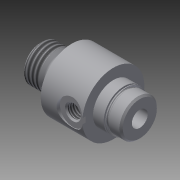
# Autodesk Inventor part: 01R000-0_rod_guide
Saved by Autodesk Inventor 2015 (Build 190159000, 159)
## iProperties
Category: PARTsolutions
Company: BIMBA
Created: 2015-01-25
Part Number: 01R000-0_rod_guide
Material: Generic
Catalog Web Link: www.cadenas.de
Description: Rod Guide-Original Line - Standard Air Cylinders
Vendor: BIMBA
Document SubType Name: Standard Catalog Part
Designer: whitaus15
Manufacturer: BIMBA
Mass: 4.50765 g
Surface Area: 24.6874 cm^2
Volume: 4.50765 cm^3
Density: 1 g/cm^3
Appearance: PSOLRGB-211-211-211
PSOL_IDENT_0: {$CADENAS_DATA\23d-libs\bimba\bimba\bimba_imperial\bimba_full_line\original_line_cylinders\standard_
PSOL_IDENT_1: air_cylinders\rod_guide.prj},232 {VTYP=3D},{NB=01R000-0_rod_guide},{LINA=01R000-0_rod_guide},{NN=Rod
PSOL_IDENT_2: Guide},{DATE=05.09.2013 09:10:53},{GEOMDATE=05.09.2013 11:10:00},{VERSION=},{LINEID=20},{LINESUBID=
PSOL_IDENT_3: -1},{WBVAR=MNT,ACTING,NR,K,Q,T1,T2,T3,T4,MB,TRIM,CUSH,RODTRANS}  {NB=01R000-0_rod_guide},{LINA=01R00
PSOL_IDENT_4: 0-0_rod_guide},{KT=DUMMY},{PN=01R000},{BORE=0.43750000},{BOREPN=01},{MNT=},{MNTALG='' , 'Front Nose'
PSOL_IDENT_5: , 'BF' , 'Front Block' , 'BFT' , 'Front Trunnion'},{ACTING=R},{ACTINGALG= '' , 'Single Acting' , 'R'
PSOL_IDENT_6: , 'Reverse/Double Acting' },{NR=},{NRALG= '' , 'N/A' },{K=},{Q=},{QALG= '' , 'Without Side Ported R
PSOL_IDENT_7: ear Head' , 'Q' , 'With Side Ported Rear Head' },{T1=},{T2=},{T3=},{T4=},{MB=0},{A1=1.1880},{A1N=0.6
PSOL_IDENT_8: 880},{A1P=1.1880},{A1B=1.1880},{A2=0.3750},{A2N=0.3130},{A2P=0.3750},{A3=0.6250},{A3N=0.1250},{A3P=0
PSOL_IDENT_9: .6250},{A4=0.1880},{A4N=0.2500},{A4P=0.1880},{A5=0.0200},{A6=0.0000},{A6N=0.0620},{A6P=0.0000},{A7=0
PSOL_IDENT_10: .5940},{A7N=0.1880},{A7P=0.5940},{A8=0.0200},{A8N=0.0200},{A8NR=0.0200},{D1=0.7380},{D1N=0.4840},{D1
PSOL_IDENT_11: P=0.7380},{D1B=0.0000},{D2=0.4465},{D3=0.0000},{D3N=0.3470},{D3P=0.0000},{D4=0.2820},{D4N=0.2220},{D
PSOL_IDENT_12: 4P=0.2820},{D4NR=0.2820},{D5=0.1895},{D5N=0.1895},{D5NR=0.1895},{C1=0.000},{C2=0.0200},{C2N=0.0200},
PSOL_IDENT_13: {C2P=0.0200},{C3=0.0000},{C3N=0.0000},{C3P=0.0000},{C4=0.0000},{C4N=0.0000},{C4P=0.0000},{NDM=0.4375
PSOL_IDENT_14: },{NDMN=0.3750},{NDMP=0.4375},{TAB=UNF},{D6=0.4350},{D6N=0.3725},{D6P=0.4350},{A9=0.0475},{A9N=0.050
PSOL_IDENT_15: 0},{A9P=0.0475},{D7=0.3600},{D7N=0.3100},{D7P=0.3600},{A10=0.0775},{A10N=0.0655},{A10P=0.0775},{R1=0
PSOL_IDENT_16: .0315},{R1N=0.0265},{R1P=0.0315},{D8=0.0000},{D9=0.0000},{D10=0.0000},{A11=0.0000},{A12=0.0000},{A13=
PSOL_IDENT_17: 0.0000},{A14=0.4680},{A14N=0.4680},{A14B=0.4690},{D11=0.0000},{D11N=0.0000},{NDM2=0.1900},{NDM2N=0.1
PSOL_IDENT_18: 900},{NDM2DP=0.0000},{THREAD=0},{HEX=0.1920},{HEXN=0.1920},{S1=0.7500},{B1=0.1275},{B2=0.3120},{B22=
PSOL_IDENT_19: 0.4380},{DB=0.3020},{B3=0.2200},{B4=0.4380},{X1=0.0620},{X2=0.4345},{NDM3=0.1640},{NDM4=0.1640},{NDM
PSOL_IDENT_20: 4DP=0.2500},{DD=0.7500},{CB=0.0000},{CBDP=0.0000},{PORT=1},{XT=0.3120},{XTX=0.3120},{XT1=0.3740},{XT
PSOL_IDENT_21: 2=0.2500},{NDMH=0.0000},{OD=0.4855},{ID=0.4465},{G=0.0000},{PNUT=0.3275},{TRIM=0},{C11=0.0000},{C22=
PSOL_IDENT_22: 0.0000},{C33=0.0000},{C44=0.0000},{C55=0.0000},{CD1=0.0000},{CD2=0.0000},{CD3=0.0000},{CNDM3=0.0000}
PSOL_IDENT_23: ,{CTAB3=0.0000},{CUSH=0},{XX=0.43800},{LCD=0.0000},{RODTRANS=0.00000}
NN: Rod Guide
NT: Original Line - Standard Air Cylinders
NB: 01R000-0_rod_guide
NBSYN: $PN.-$RODTRANS._rod_guide
LINA: 01R000-0_rod_guide
BORE: 7/16
BOREPN: 01
MNT: Front Nose
MNTALG: '' , 'Front Nose' , 'BF' , 'Front Block' , 'BFT' , 'Front Trunnion'
ACTING: Reverse/Double Acting
NR: N/A
K: Standard
Q: Without Side Ported Rear Head
T1: without T1
T2: without T2
T3: without T3
T4: without T4
MB: 0
A1N: 0.6880
A1P: 1.1880
A1B: 1.1880
A2N: 0.3130
A2P: 0.3750
A3N: 0.1250
A3P: 0.6250
A4N: 0.2500
A4P: 0.1880
A5: 0.0200
A6N: 0.0620
A6P: 0.0000
A7N: 0.1880
A7P: 0.5940
A8N: 0.0200
A8NR: 0.0200
D1N: 0.4840
D1P: 0.7380
D1B: 0.0000
D2: 0.4465
D3N: 0.3470
D3P: 0.0000
D4N: 0.2220
D4P: 0.2820
D4NR: 0.2820
D5N: 0.1895
D5NR: 0.1895
C1: 0.000
C2N: 0.0200
C2P: 0.0200
C3N: 0.0000
C3P: 0.0000
C4N: 0.0000
C4P: 0.0000
NDMN: 0.3750
NDMP: 0.4375
TAB: UNF
D6N: 0.3725
D6P: 0.4350
A9N: 0.0500
A9P: 0.0475
D7N: 0.3100
D7P: 0.3600
A10N: 0.0655
A10P: 0.0775
R1N: 0.0265
R1P: 0.0315
D8: 0.0000
D9: 0.0000
D10: 0.0000
A11: 0.0000
A12: 0.0000
A13: 0.0000
A14N: 0.4680
A14B: 0.4690
D11N: 0.0000
NDM2N: 0.1900
NDM2DP: 0.0000
HEXN: 0.1920
S1: 0.7500
B1: 0.1275
B2: 0.3120
B22: 0.4380
DB: 0.3020
B3: 0.2200
B4: 0.4380
X1: 0.0620
X2: 0.4345
NDM3: 0.1640
NDM4: 0.1640
NDM4DP: 0.2500
DD: 0.7500
CB: 0.0000
CBDP: 0.0000
XTX: 0.3120
XT1: 0.3740
XT2: 0.2500
NDMH: 0.0000
TRIM: 0
C11: 0.0000
C22: 0.0000
C33: 0.0000
C44: 0.0000
C55: 0.0000
CD1: 0.0000
CD2: 0.0000
CD3: 0.0000
CNDM3: 0.0000
CTAB3: 0.0000
CUSH: 0
LCD: 0.0000
RODTRANS: 0.00000
SUPPLIER: BIMBA
ARTICLENO: 01R000-0_rod_guide
BOMINFO: 01R000-0_rod_guide
CREATOR: CADENAS GmbH
Title: 01R000-0_rod_guide
Author: Cadenas PARTsolutions
Comments: Original Line - Standard Air Cylinders
Autodesk Inventor part; units mm, degrees
sketch "Sketch_2" plane through (0, 0, 0) normal (0, 0, 1) x (1, 0, 0)
  line L0 (9.525, 0) -> (0, 0)
  line L1 (0, 0) -> (0, 4.8006)
  line L2 (0, 4.8006) -> (0.7557, 5.5563)
  line L3 (0.7557, 5.5563) -> (5.0286, 5.5563)
  line L4 (5.0286, 5.5563) -> (5.7864, 4.8042)
  arc A0 (5.7864, 4.8042) -> (6.35, 4.572) centre (6.35, 5.3721) ccw
  line L5 (6.35, 4.572) -> (7.5184, 4.572)
  arc A1 (7.5184, 4.572) -> (8.3185, 5.3721) centre (7.5184, 5.3721) ccw
  line L6 (8.3185, 5.3721) -> (8.3185, 5.5245)
  line L7 (8.3185, 5.5245) -> (9.525, 5.5245)
  line L8 (9.525, 5.5245) -> (9.525, 0)
  line L9 (9.525, 0) -> (0, 0)
  constraints: 20 end point, 4 point on circle, 2 centre point
revolve "Revolution1" add sketch "Sketch_2" angle 360 about axis through (9.525, 0, 0) along (1, 0, 0)
thread "Thread1" size "7/16-20 UNF" class "2A" standard "ANSI Unified Screw Threads" full length
sketch "Sketch_3" plane through (0, 0, 0) normal (0, 0, 1) x (1, 0, 0)
  line L0 (30.1752, 0) -> (9.525, 0)
  line L1 (9.525, 0) -> (9.525, 9.3726)
  line L2 (9.525, 9.3726) -> (25.4, 9.3726)
  line L3 (25.4, 9.3726) -> (25.4, 5.1626)
  line L4 (25.4, 5.1626) -> (25.908, 5.1626)
  line L5 (25.908, 5.1626) -> (26.416, 5.6706)
  line L6 (26.416, 5.6706) -> (29.6672, 5.6706)
  line L7 (29.6672, 5.6706) -> (30.1752, 5.1626)
  line L8 (30.1752, 5.1626) -> (30.1752, 0)
  line L9 (30.1752, 0) -> (9.525, 0)
  constraints: 20 end point
revolve "Revolution2" add sketch "Sketch_3" angle 360 about axis through (30.1752, 0, 0) along (1, 0, 0)
sketch "Sketch3" plane through (0, 0, 0) normal (-1, 0, 0) x (0, 0, 1)
  point P0 (0, 0)
hole "Hole1" at (0, 0, 0) direction (1, 0, 0) diameter 4.8133 depth 30.1752 countersink diameter 5.8293 countersink angle 90
sketch "Sketch_12" plane through (0, 0, 0) normal (0, 1, 0) x (-1, 0, 0)
  line L0 (-18.288, 9.3726) -> (-18.288, -1.016)
  line L1 (-18.288, -1.016) -> (-20.2717, -1.016)
  line L2 (-20.2717, -1.016) -> (-20.2717, 7.9273)
  line L3 (-20.2717, 7.9273) -> (-20.701, 8.3566)
  line L4 (-20.701, 8.3566) -> (-22.2504, 8.3566)
  line L5 (-22.2504, 8.3566) -> (-22.2504, 9.3726)
  line L6 (-22.2504, 9.3726) -> (-18.288, 9.3726)
  line L7 (-18.288, 9.3726) -> (-18.288, -1.016)
  constraints: 16 end point
revolve "Revolution3" cut sketch "Sketch_12" angle 360 about axis through (18.288, 0, 9.3726) along (0, 0, 1)
thread "Thread2" size "10-32 UNF" class "2B" standard "ANSI Unified Screw Threads" length 4.7752 offset 2.2188
sketch "Sketch_14" plane through (0, 0, 0) normal (0, 0, 1) x (1, 0, 0)
  line L0 (25.4, 0) -> (22.1615, 0)
  line L1 (22.1615, 6.1659) -> (25.4, 6.1659)
  line L2 (25.4, 6.1659) -> (25.4, 9.9758)
  line L3 (25.4, 9.9758) -> (22.1615, 9.9758)
  line L4 (22.1615, 9.9758) -> (22.1615, 6.1659)
  constraints: 10 end point
revolve "Revolution4" cut sketch "Sketch_14" angle 360 about axis through (25.4, 0, 0) along (1, 0, 0)
sketch "Sketch_47" plane through (0, 0, 0) normal (0, 0, 1) x (1, 0, 0)
  line L0 (25.908, 0) -> (25.4, 0)
  line L1 (25.4, 4.9085) -> (25.908, 4.9085)
  line L2 (25.908, 4.9085) -> (25.908, 5.1626)
  line L3 (25.908, 5.1626) -> (25.654, 5.1626)
  line L4 (25.654, 5.1626) -> (25.5116, 5.305)
  arc A0 (25.5116, 5.4846) -> (25.5116, 5.305) centre (25.6014, 5.3948) ccw
  line L5 (25.5116, 5.4846) -> (26.1087, 6.0817)
  line L6 (26.1087, 6.0817) -> (26.1087, 6.1659)
  line L7 (26.1087, 6.1659) -> (25.9055, 6.1659)
  line L8 (25.9055, 6.1659) -> (25.4, 5.6603)
  line L9 (25.4, 5.6603) -> (25.4, 4.9085)
  constraints: 20 end point, 2 point on circle, 1 centre point
revolve "Revolution5" add sketch "Sketch_47" angle 360 about axis through (25.908, 0, 0) along (1, 0, 0)
ref_plane "dp1_XY" through (9.525, 5.5245, 0) normal (0, 0, 1) x (1, 0, 0)
ref_plane "dp1_YZ" through (9.525, 5.5245, 0) normal (1, 0, 0) x (0, 1, 0)
ref_plane "dp1_ZX" through (9.525, 5.5245, 0) normal (0, 1, 0) x (0, 0, 1)
ref_plane "dp2_XY" through (9.525, -5.5245, 0) normal (0, 0, 1) x (1, 0, 0)
ref_plane "dp2_YZ" through (9.525, -5.5245, 0) normal (1, 0, 0) x (0, 1, 0)
ref_plane "dp2_ZX" through (9.525, -5.5245, 0) normal (0, 1, 0) x (0, 0, 1)
ref_plane "port_XY" through (18.288, 0, 0) normal (0, 0, 1) x (1, 0, 0)
ref_plane "port_YZ" through (18.288, 0, 0) normal (1, 0, 0) x (0, 1, 0)
ref_plane "port_ZX" through (18.288, 0, 0) normal (0, 1, 0) x (0, 0, 1)
ref_plane "rod_guide_XY" through (0, 0, 0) normal (1, 0, 0) x (0, 0, -1)
ref_plane "rod_guide_YZ" through (0, 0, 0) normal (0, 0, -1) x (0, 1, 0)
ref_plane "rod_guide_ZX" through (0, 0, 0) normal (0, 1, 0) x (1, 0, 0)
ref_plane "s1_XY" through (8.3185, 0, 0) normal (0, 0, 1) x (1, 0, 0)
ref_plane "s1_YZ" through (8.3185, 0, 0) normal (1, 0, 0) x (0, 1, 0)
ref_plane "s1_ZX" through (8.3185, 0, 0) normal (0, 1, 0) x (0, 0, 1)
ref_plane "s2_XY" through (9.525, 0, 0) normal (0, 0, 1) x (1, 0, 0)
ref_plane "s2_YZ" through (9.525, 0, 0) normal (1, 0, 0) x (0, 1, 0)
ref_plane "s2_ZX" through (9.525, 0, 0) normal (0, 1, 0) x (0, 0, 1)
ref_plane "t1_XY" through (9.525, 0, 0) normal (1, 0, 0) x (0, 0, -1)
ref_plane "t1_YZ" through (9.525, 0, 0) normal (0, 0, -1) x (0, 1, 0)
ref_plane "t1_ZX" through (9.525, 0, 0) normal (0, 1, 0) x (1, 0, 0)
ref_plane "t111_XY" through (9.525, 0, 0) normal (1, 0, 0) x (0, 0, -1)
ref_plane "t111_YZ" through (9.525, 0, 0) normal (0, 0, -1) x (0, 1, 0)
ref_plane "t111_ZX" through (9.525, 0, 0) normal (0, 1, 0) x (1, 0, 0)
ref_plane "to_foot_bracket_XY" through (9.525, 0, 0) normal (1, 0, 0) x (0, 0, -1)
ref_plane "to_foot_bracket_YZ" through (9.525, 0, 0) normal (0, 0, -1) x (0, 1, 0)
ref_plane "to_foot_bracket_ZX" through (9.525, 0, 0) normal (0, 1, 0) x (1, 0, 0)
ref_plane "to_nut_XY" through (8.3185, 0, 0) normal (1, 0, 0) x (0, 0, -1)
ref_plane "to_nut_YZ" through (8.3185, 0, 0) normal (0, 0, -1) x (0, 1, 0)
ref_plane "to_nut_ZX" through (8.3185, 0, 0) normal (0, 1, 0) x (1, 0, 0)
ref_plane "to_rod_XY" through (0, 0, 0) normal (1, 0, 0) x (0, 0, -1)
ref_plane "to_rod_YZ" through (0, 0, 0) normal (0, 0, -1) x (0, 1, 0)
ref_plane "to_rod_ZX" through (0, 0, 0) normal (0, 1, 0) x (1, 0, 0)
ref_plane "to_screw_XY" through (18.288, 0, 0) normal (0, 1, 0) x (1, 0, 0)
ref_plane "to_screw_YZ" through (18.288, 0, 0) normal (1, 0, 0) x (0, 0, -1)
ref_plane "to_screw_ZX" through (18.288, 0, 0) normal (0, 0, -1) x (0, 1, 0)
ref_plane "to_trunnion_brackets_XY" through (7.9248, 0, 0) normal (0, 1, 0) x (1, 0, 0)
ref_plane "to_trunnion_brackets_YZ" through (7.9248, 0, 0) normal (1, 0, 0) x (0, 0, -1)
ref_plane "to_trunnion_brackets_ZX" through (7.9248, 0, 0) normal (0, 0, -1) x (0, 1, 0)
ref_plane "to_trunnion_brackets1_XY" through (7.9248, 9.525, 0) normal (0, 1, 0) x (1, 0, 0)
ref_plane "to_trunnion_brackets1_YZ" through (7.9248, 9.525, 0) normal (1, 0, 0) x (0, 0, -1)
ref_plane "to_trunnion_brackets1_ZX" through (7.9248, 9.525, 0) normal (0, 0, -1) x (0, 1, 0)
ref_plane "to_trunnion_brackets2_XY" through (7.9248, -9.525, 0) normal (0, 1, 0) x (1, 0, 0)
ref_plane "to_trunnion_brackets2_YZ" through (7.9248, -9.525, 0) normal (1, 0, 0) x (0, 0, -1)
ref_plane "to_trunnion_brackets2_ZX" through (7.9248, -9.525, 0) normal (0, 0, -1) x (0, 1, 0)
ref_plane "to_tube_XY" through (25.908, 0, 0) normal (1, 0, 0) x (0, 0, -1)
ref_plane "to_tube_YZ" through (25.908, 0, 0) normal (0, 0, -1) x (0, 1, 0)
ref_plane "to_tube_ZX" through (25.908, 0, 0) normal (0, 1, 0) x (1, 0, 0)
body "Solid1"
